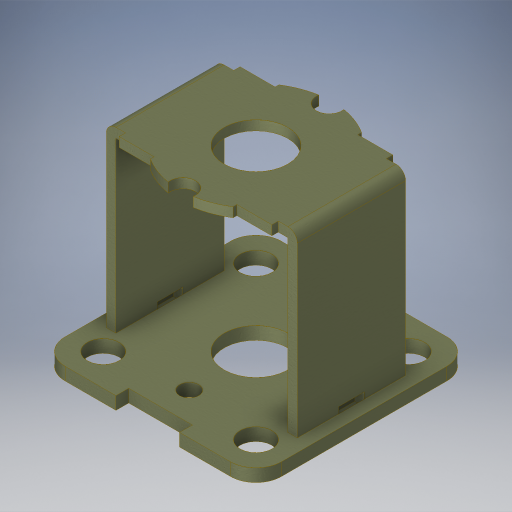
# Autodesk Inventor part: Frame
Saved by Autodesk Inventor 2024.1 (Build 281209000, 209)
## iProperties
Created: 2019-04-29
Part Number: Frame
Material: Steel, Galvanized
Document SubType Name: Sheet Metal
Designer: Plo
Density: 7.85 g/cm^3
Sheet Metal Rule: Default_mm
Appearance: Gold
Author: Plo
Autodesk Inventor part; units mm, degrees
ref_plane "YZ Plane" through (0, 0, 0) normal (1, 0, 0) x (0, 1, 0)
ref_plane "XZ Plane" through (0, 0, 0) normal (0, 1, 0) x (-1, 0, 0)
ref_plane "XY Plane" through (0, 0, 0) normal (0, 0, 1) x (1, 0, 0)
sketch "Sketch1" plane through (0, 0, 0) normal (0, 1, 0) x (-1, 0, 0)
  line L0 (-9.5, 15) -> (9.5, 15)
  line L1 (9.5, -15) -> (-9.5, -15)
  line L2 (-9.5, 15) -> (9.5, -15) construction
  line L3 (9.5, 15) -> (-9.5, -15) construction
  arc A0 (11.837, 1.9714) -> (11.837, -1.9714) centre (11.5, 0) ccw
  arc A1 (-11.837, -1.9714) -> (-11.837, 1.9714) centre (-11.5, 0) ccw
  arc A2 (11.837, 1.9714) -> (9.5, 7.3314) centre (0, 0) ccw
  arc A3 (-9.5, 7.3314) -> (-11.837, 1.9714) centre (0, 0) ccw
  arc A4 (-11.837, -1.9714) -> (-9.5, -7.3314) centre (0, 0) ccw
  arc A5 (9.5, -7.3314) -> (11.837, -1.9714) centre (0, 0) ccw
  line L4 (9.5, 15) -> (9.5, 6.5)
  line L5 (9.5, -6.5) -> (9.5, -15)
  line L6 (-9.5, -15) -> (-9.5, -6.5)
  line L7 (-9.5, 6.5) -> (-9.5, 15)
  circle A6 centre (0, 0) radius 5
  line L8 (9.5, -12) -> (8.5, -12)
  line L9 (8.5, -12) -> (8.5, -15)
  line L10 (8.5, -15) -> (9.5, -15)
  line L11 (9.5, -15) -> (9.5, -12)
  line L12 (-8.5, -15) -> (-9.5, -15)
  line L13 (-9.5, -15) -> (-9.5, -12)
  line L14 (-9.5, -12) -> (-8.5, -12)
  line L15 (-8.5, -12) -> (-8.5, -15)
  line L16 (9.5, 12) -> (8.5, 12)
  line L17 (8.5, 12) -> (8.5, 15)
  line L18 (8.5, 15) -> (9.5, 15)
  line L19 (9.5, 15) -> (9.5, 12)
  line L20 (-8.5, 15) -> (-9.5, 15)
  line L21 (-9.5, 15) -> (-9.5, 12)
  line L22 (-9.5, 12) -> (-8.5, 12)
  line L23 (-8.5, 12) -> (-8.5, 15)
  line L24 (14.0753, 6.5) -> (-14.0753, 6.5)
  line L25 (-14.0753, 6.5) -> (-14.0753, -6.5)
  line L26 (-14.0753, -6.5) -> (14.0753, -6.5)
  line L27 (14.0753, -6.5) -> (14.0753, 6.5)
  line L28 (14.0753, 6.5) -> (-14.0753, -6.5) construction
  line L29 (-14.0753, 6.5) -> (14.0753, -6.5) construction
  point P0 (0, 0)
  point P1 (9.5, 11.1657)
  point P2 (0, -15)
  point P3 (0, 15)
  point P4 (0, 0)
  point P5 (9, -12)
  point P6 (-10.0871, 6.5)
  point P7 (-10.0871, -6.5)
  point P8 (10.0871, -6.5)
  point P9 (10.0871, 6.5)
  dimension "d0" = 19
  dimension "d1" = 30
  dimension "d2" = 4
  dimension "d3" = 4
  dimension "d17" = 10
  dimension "d21" = 19
  dimension "d22" = 15
  dimension "d23" = 12
  dimension "d24" = 12
  dimension "d25" = 12
  dimension "d26" = 12
  dimension "d27" = 11.5
  dimension "d28" = 11.5
  dimension "d29" = 17
  dimension "d30" = 8.5
  dimension "d31" = 12
  dimension "d32" = 12
  dimension "d33" = 13
  constraints: 60 end point, 19 point on line, 15 parallel, 12 point on circle, 7 centre point, 7 midpoint, 7 perpendicular, 6 horizontal, 2 coincident, 2 collinear, 2 horizontal alignment, 2 vertical alignment
  measures "d0" distance of L2.end L3.end
  measures "d1" distance of L0.end L2.end
  measures "d2" diameter of A0
  measures "d3" diameter of A1
  measures "d17" diameter of A6
  measures "d21" distance from line of point (9.5, 11.166) L7
  measures "d22" distance from line of point (0, 0) L1
  measures "d23" radius of A5
  measures "d24" radius of A4
  measures "d25" radius of A2
  measures "d26" radius of A3
  measures "d27" distance of point (0, 0) A0.centre
  measures "d28" distance of A1.centre A6.centre
  measures "d29" distance between parallel lines of L15 L9
  measures "d30" distance from line of point (0, 0) L9
  measures "d31" vertical distance of A5.centre point (9, -12)
  measures "d32" distance from line of point (0, 0) L16
  measures "d33" distance of L24.end L25.end
extrude "Extrusion1" add sketch "Sketch1" along normal blind 1.5 contours L0 L17 L16 L4 L24 L7 L22 L23 | L24 A2 A0 A5 L26 A4 A1 A3 | L6 L26 L5 L8 L9 L1 L15 L14
sketch "Sketch2" plane through (-9.5, 0, 15) normal (0, 0, 1) x (1, 0, 0)
  line L0 (7.5, -28.5) -> (7.5, -26.5)
  line L1 (11.5, -28.5) -> (11.5, -26.5)
  line L2 (7.5, -26.5) -> (11.5, -26.5)
  line L3 (1, 1.5) -> (18, 1.5)
  line L4 (18, 1.5) -> (18, -28.5)
  line L5 (18, -28.5) -> (1, -28.5)
  line L6 (1, -28.5) -> (1, 1.5)
  line L7 (18, 0) -> (18, 1.5) projected
  line L8 (18, -28.5) -> (14.5, -28.5)
  line L9 (14.5, -28.5) -> (14.5, -26.5)
  line L10 (14.5, -26.5) -> (18, -26.5)
  line L11 (18, -26.5) -> (18, -28.5)
  line L12 (1, -28.5) -> (4.5, -28.5)
  line L13 (4.5, -28.5) -> (4.5, -26.5)
  line L14 (4.5, -26.5) -> (1, -26.5)
  line L15 (1, -26.5) -> (1, -28.5)
  line L16 (1, 0) -> (1, 1.5) projected
  line L17 (7.5, -26.5) -> (11.5, -26.5)
  line L18 (11.5, -26.5) -> (11.5, -25.5)
  line L19 (11.5, -25.5) -> (7.5, -25.5)
  line L20 (7.5, -25.5) -> (7.5, -26.5)
  line L21 (7.5, -28.5) -> (11.5, -28.5)
  line L22 (11.5, -28.5) -> (11.5, -27.5)
  line L23 (11.5, -27.5) -> (7.5, -27.5)
  line L24 (7.5, -27.5) -> (7.5, -28.5)
  point P0 (9.5, 1.5)
  point P1 (9.5, -26.5)
  dimension "d36" = 30
  dimension "d37" = 4
  dimension "d38" = 2
  dimension "d39" = 3
  dimension "d40" = 3
  dimension "d48" = 1
  dimension "d49" = 1
  constraints: 46 end point, 10 parallel, 7 perpendicular, 5 horizontal, 4 midpoint, 3 collinear, 2 point on line, 1 vertical alignment
  measures "d36" distance of L3.end L4.end
  measures "d37" distance of L0.end L1.end
  measures "d38" distance between parallel lines of L5 L2
  measures "d39" distance between parallel lines of L0 L13
  measures "d40" distance between parallel lines of L9 L1
  measures "d48" distance of L19.end L0.end
  measures "d49" distance between parallel lines of L21 L23
extrude "Extrusion2" add sketch "Sketch2" against normal blind 1.5 contours L5 L13 L14 L6 L3 L4 L10 L9 L1 L18 L19 L20 L0 | L0 L23 L1 L5
mirror "Mirror2" about plane through (0, 0, 0) normal (0, 0, 1) of "Extrusion2"
fillet "Fillet1" radius 1.5 2 edges at (0, 1.5, 15) (0, 1.5, -15)
sketch "Sketch4" plane through (2, -28.5, 15) normal (0, -1, 0) x (1, 0, 0)
  line L0 (-19, -32) -> (15, -32)
  line L1 (15, -32) -> (15, 2)
  line L2 (15, 2) -> (-19, 2)
  line L3 (-19, 2) -> (-19, -32)
  line L4 (-19, -32) -> (15, 2) construction
  line L5 (15, -32) -> (-19, 2) construction
  point P0 (-2, -15)
  dimension "d44" = 34
  dimension "d45" = 34
  constraints: 12 end point, 2 midpoint, 2 parallel, 1 horizontal, 1 perpendicular
  measures "d44" distance of L0.end L1.end
  measures "d45" distance of L1.end L2.end
extrude "Extrusion3" add sketch "Sketch4" against normal blind 2 separate body
sketch "Sketch5" plane through (2, -28.5, 15) normal (0, -1, 0) x (1, 0, 0)
  line L0 (-14, -27) -> (10, -27)
  line L1 (10, -27) -> (10, -3)
  line L2 (10, -3) -> (-14, -3)
  line L3 (-14, -3) -> (-14, -27)
  line L4 (-14, -27) -> (10, -3) construction
  line L5 (10, -27) -> (-14, -3) construction
  point P0 (-2, -15)
  dimension "d50" = 24
  dimension "d51" = 24
  constraints: 12 end point, 2 midpoint, 2 parallel, 1 horizontal, 1 perpendicular
  measures "d50" distance of L0.end L1.end
  measures "d51" distance of L1.end L2.end
hole "Hole1" at (-12, -28.5, 12) at (12, -28.5, 12) at (12, -28.5, -12) at (-12, -28.5, -12) direction (0, 1, 0) diameter 5 end through all bodies 2
fillet "Fillet2" radius 4 4 edges at (17, -27.5, 17) (-17, -27.5, 17) (-17, -27.5, -17) (17, -27.5, -17)
sketch "Sketch6" plane through (2, -28.5, 15) normal (0, -1, 0) x (1, 0, 0)
  line L0 (-7, 0) -> (3, 0) projected
  line L1 (-7, 0) -> (-7, -1.5) projected
  line L2 (3, -1.5) -> (-7, -1.5) projected
  line L3 (3, 0) -> (3, -1.5) projected
  line L4 (-7, -30) -> (3, -30) projected
  line L5 (3, -30) -> (3, -28.5) projected
  line L6 (3, -28.5) -> (-7, -28.5) projected
  line L7 (-7, -30) -> (-7, -28.5) projected
  point P0 (-2, -15)
extrude "Extrusion4" cut sketch "Sketch6" against normal through all bodies 2
sketch "Sketch7" plane through (2, -28.5, 15) normal (0, -1, 0) x (1, 0, 0)
  line L0 (-7, -30) -> (3, -30) projected
  line L1 (3, -30) -> (3, -28.5) projected
  line L2 (3, -28.5) -> (-7, -28.5) projected
  line L3 (-7, -28.5) -> (-7, -30) projected
  line L4 (-7, 0) -> (-7, -1.5) projected
  line L5 (-7, -1.5) -> (3, -1.5) projected
  line L6 (3, -1.5) -> (3, 0) projected
  line L7 (3, 0) -> (-7, 0) projected
  arc A0 (-19, -28) -> (-15, -32) centre (-15, -28) ccw projected
  line L8 (-19, -28) -> (-19, -2) projected
  arc A1 (-15, 2) -> (-19, -2) centre (-15, -2) ccw projected
  line L9 (-15, 2) -> (11, 2) projected
  arc A2 (15, -2) -> (11, 2) centre (11, -2) ccw projected
  line L10 (15, -2) -> (15, -28) projected
  arc A3 (11, -32) -> (15, -28) centre (11, -28) ccw projected
  line L11 (11, -32) -> (-15, -32) projected
  circle A4 centre (-14, -27) radius 2.5 projected
  circle A5 centre (10, -27) radius 2.5 projected
  circle A6 centre (10, -3) radius 2.5 projected
  circle A7 centre (-14, -3) radius 2.5 projected
  line L12 (-19, -10) -> (-17, -10)
  line L13 (-17, -10) -> (-17, -20)
  line L14 (-17, -20) -> (-19, -20)
  line L15 (-19, -20) -> (-19, -10)
  line L16 (15, -10) -> (13, -10)
  line L17 (13, -10) -> (13, -20)
  line L18 (13, -20) -> (15, -20)
  line L19 (15, -20) -> (15, -10)
  point P0 (-2, -15)
  point P1 (-19, -15)
  point P2 (15, -20)
  dimension "d62" = 2
  dimension "d63" = 2
  dimension "d64" = 10
  constraints: 16 end point, 4 parallel, 3 point on line, 2 horizontal, 2 midpoint, 2 perpendicular, 1 collinear
  measures "d62" distance of L16.start L16.end
  measures "d63" distance of L12.start L12.end
  measures "d64" distance of L12.end L13.end
extrude "Extrusion5" cut sketch "Sketch7" against normal through all contours L8 L12 L13 L14 | L18 L17 L16 L10 bodies 2
sketch "Sketch8" plane through (2, -28.5, 15) normal (0, -1, 0) x (1, 0, 0)
  circle A0 centre (-2, -15) radius 5 projected
  point P0 (-2, -15)
extrude "Extrusion6" cut sketch "Sketch8" against normal through all bodies 2
sketch "Sketch9" plane through (2, -28.5, 15) normal (0, -1, 0) x (1, 0, 0)
  line L0 (-12.5, -15) -> (8.5, -15)
  line L1 (11, 2) -> (-15, 2) projected
  point P0 (-2, -15)
  point P1 (-2, -15)
  dimension "d69" = 21
  constraints: 2 end point, 1 coincident, 1 midpoint, 1 parallel
  measures "d69" distance of L0.start L0.end
hole "Hole2" at (-10.5, -28.5, 0) at (10.5, -28.5, 0) direction (0, 1, 0) diameter 3 end through all bodies 2
equation "\"d21\" = d0"
equation "\"d22\" = 0.5 * d1"
equation "\"d28\" = d27"
equation "\"d30\" = 0.5 * d29"
equation "\"d32\" = d31"
equation "\"d40\" = d39"
equation "\"d45\" = d44"
equation "\"d57\" = Thickness"
equation "\"d63\" = d62"
equation "\"BendReliefWidth\" = Thickness"
equation "\"BendReliefDepth\" = 0.5 * Thickness"
equation "\"CornerReliefSize\" = 4 * Thickness"
equation "\"MinimumRemnant\" = 2 * Thickness"
equation "\"GapSize\" = Thickness"
equation "\"d4\" = Thickness"
equation "\"Thickness\" = 1.5"
body "Solid1"
body "Solid2"
